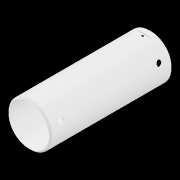
# Autodesk Inventor part: right_hull_mid
Saved by Autodesk Inventor 2020.2 (Build 242310000, 310)
## iProperties
Created: 2019-11-08
Part Number: right_hull_mid
Material: PVC-Piping
Document SubType Name: Modeling
Designer: agmle
Mass: 4504.18 g
Surface Area: 7642.52 cm^2
Volume: 3217.27 cm^3
Density: 1.4 g/cm^3
Appearance: Smooth - White
Author: agmle
Autodesk Inventor part; units mm, degrees
ref_plane "YZ Plane" through (0, 0, 0) normal (1, 0, 0) x (0, 1, 0)
sketch "Sketch1" plane through (0, 0, 0) normal (0, 0, 1) x (1, 0, 0)
  circle A0 centre (0, 0) radius 109.5375
  circle A1 centre (0, 0) radius 100.8634
  dimension "d0" = 219.075
  dimension "d1" = 8.6741
  constraints: 2 centre point, 2 coincident
  measures "d0" diameter of A0
  measures "d1" radial gap between concentric circles of A0 A1
extrude "PVC Pipe" add sketch "Sketch1" along normal blind 609.6
sketch "Sketch2" plane through (0, 0, 0) normal (0, 0, -1) x (-1, 0, 0)
  line L0 (-74.8665, 79.9592) -> (-109.5375, 79.9592)
  line L1 (-109.5375, 79.9592) -> (-109.5375, -79.9592)
  line L2 (-109.5375, -79.9592) -> (-74.8665, -79.9592)
  line L3 (-74.8665, -79.9592) -> (-74.8665, 79.9592)
  circle A0 centre (0, 0) radius 109.5375 construction
  dimension "d4" = 34.671
  constraints: 8 end point, 2 parallel, 2 point on circle, 1 horizontal, 1 perpendicular, 1 tangent
  measures "d4" distance of L0.start L0.end
extrude "Drive Deck" cut sketch "Sketch2" against normal blind 152.4
chamfer "Sealant Surface" distance 8.6741 angle 45 2 edges at (-109.5375, 0, 609.6) (-109.5375, 0, 0)
ref_plane "Work Plane1" through (0, 109.5375, 0) normal (0, 1, 0) x (-1, 0, 0)
sketch "Sketch3" plane through (0, 109.5375, 0) normal (0, 1, 0) x (-1, 0, 0)
  line L0 (-100.8634, 609.6) -> (100.8634, 609.6) construction
  line L1 (-74.8665, 0) -> (100.8634, 0) construction
  line L2 (41.8167, 550.1259) -> (41.8167, 59.4741) construction
  line L3 (109.5375, 8.6741) -> (109.5375, 600.9259) construction
  line L4 (41.8167, 304.8) -> (109.5375, 304.8) construction
  line L5 (109.5375, 600.9259) -> (-109.5375, 600.9259) construction
  point P0 (0, 0)
  dimension "d11" = 41.8167
  dimension "d13" = 50.8
  constraints: 4 end point, 2 midpoint, 1 perpendicular, 1 vertical
  measures "d11" distance from line of point (0, 0) L2
  measures "d13" distance from line of L5 L2.start
hole "Cable Ports" at (-41.8167, 109.5375, 550.1259) at (-41.8167, 109.5375, 59.4741) direction (0, -1, 0) diameter 26.6446 end up to surface
fillet "Cable Softening" radius 3.175 2 edges at (-42.7148, 91.3722, 536.8339) (-42.7148, 91.3722, 46.1821)
ref_plane "Work Plane2" through (-109.5375, 0, 0) normal (1, 0, 0) x (0, 1, 0)
sketch "Sketch4" plane through (-109.5375, 0, 0) normal (1, 0, 0) x (0, 1, 0)
  line L0 (-38.1, 53.1241) -> (38.1, 53.1241)
  line L1 (38.1, 53.1241) -> (38.1, 34.0741)
  line L2 (38.1, 34.0741) -> (-38.1, 34.0741)
  line L3 (-38.1, 34.0741) -> (-38.1, 53.1241)
  line L4 (-109.5375, 8.6741) -> (109.5375, 8.6741) projected
  point P0 (0, 0)
  point P1 (-79.9592, 8.6741)
  point P2 (79.9592, 8.6741)
  point P3 (0, 34.0741)
  dimension "d22" = 76.2
  dimension "d23" = 19.05
  dimension "d24" = 25.4
  constraints: 8 end point, 2 parallel, 1 horizontal, 1 midpoint, 1 perpendicular, 1 vertical alignment
  measures "d22" distance of L1.end L2.end
  measures "d23" distance of L0.end L1.end
  measures "d24" distance between parallel lines of L4 L2
extrude "Piercing Flats" cut sketch "Sketch4" along normal blind 6.35
sketch "Sketch5" plane through (-103.1875, 0, 0) normal (-1, 0, 0) x (0, 0, 1)
  line L0 (53.1241, -36.7533) -> (53.1241, 36.7533) construction
  line L1 (53.1241, 0) -> (34.0741, 0) construction
  line L2 (34.0741, 36.7533) -> (34.0741, -36.7533) construction
  point P0 (0, 0)
  point P1 (43.5991, 0)
  constraints: 3 midpoint, 2 end point
hole "Winch Gland" at (-103.1875, 0, 43.5991) direction (1, 0, 0) diameter 12.7 end through all
equation "\"d0\" = hull_od"
equation "\"d1\" = hull_wall"
equation "\"d2\" = hull_length"
equation "\"d4\" = slab_thick"
equation "\"d5\" = 2 * impeller_od"
equation "\"d8\" = hull_wall"
equation "\"d11\" = strut_hole_offset"
equation "\"d14\" = conduit_od - 2 * conduit_wall_thick"
equation "\"hull_od\" = 219.075"
equation "\"hull_id\" = 201.7268"
equation "\"hull_wall\" = 8.6741"
equation "\"hull_length\" = 609.6"
equation "\"hull_spacing\" = 390.525"
equation "\"impeller_od\" = 76.2"
equation "\"impeller_clearance\" = 0.5"
equation "\"impeller_shaft_id\" = 3.175"
equation "\"impeller_shaft_od\" = 5.715"
equation "\"impeller_shaft_support\" = 3.175"
equation "\"impeller_intake_od\" = 19.05"
equation "\"impeller_vane_thick\" = 2"
equation "\"impeller_vane_inner_rad\" = 3.175"
equation "\"impeller_vane_outer_rad\" = 0.37206"
equation "\"magnet_od\" = 5.95"
equation "\"magnet_clearance\" = 0.25"
equation "\"magnet_rad\" = 0.25"
equation "\"magnet_circle_offset\" = 3.175"
equation "\"motor_shaft_od\" = 12.7"
equation "\"motor_shaft_length\" = 31.75"
equation "\"motor_shaft_key\" = 3.048"
equation "\"slab_thick\" = 34.671"
equation "\"conduit_od\" = 29.5402"
equation "\"conduit_wall_thick\" = 1.4478"
equation "\"strut_hole_offset\" = 41.81674"
body "Solid1"
